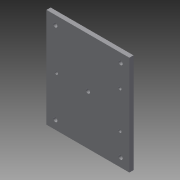
# Autodesk Inventor part: small plate
Saved by Autodesk Inventor 2014 SP1 (Build 180222100, 222)
## iProperties
Created: 2014-02-07
Part Number: small plate
Material: Generic
Document SubType Name: Modeling
Designer: Owner
Density: 1 g/cm^3
Appearance: Default
Author: Owner
Autodesk Inventor part; units mm, degrees
ref_plane "YZ Plane" through (0, 0, 0) normal (1, 0, 0) x (0, 1, 0)
ref_plane "XZ Plane" through (0, 0, 0) normal (0, 1, 0) x (-1, 0, 0)
ref_plane "XY Plane" through (0, 0, 0) normal (0, 0, 1) x (1, 0, 0)
sketch "Sketch1" plane through (0, 0, 0) normal (0, 0, 1) x (1, 0, 0)
  line L0 (-63.5, -76.2) -> (63.5, -76.2)
  line L1 (63.5, -76.2) -> (63.5, 76.2)
  line L2 (63.5, 76.2) -> (-63.5, 76.2)
  line L3 (-63.5, 76.2) -> (-63.5, -76.2)
  line L4 (-63.5, -76.2) -> (63.5, 76.2) construction
  line L5 (63.5, -76.2) -> (-63.5, 76.2) construction
  line L6 (-63.5, 76.2) -> (-50.0296, 62.7296)
  line L7 (-63.5, 76.2) -> (-44.45, 76.2) construction
  line L8 (63.5, 76.2) -> (69.85, 76.2) construction
  line L9 (63.5, 76.2) -> (50.0296, 62.7296)
  line L10 (63.5, -76.2) -> (50.0296, -62.7296)
  line L11 (-63.5, -76.2) -> (-50.0296, -62.7296)
  circle A0 centre (-50.0296, 62.7296) radius 3.175
  circle A1 centre (50.0296, 62.7296) radius 3.175
  circle A2 centre (50.0296, -62.7296) radius 3.175
  circle A3 centre (-50.0296, -62.7296) radius 3.175
  circle A4 centre (0, 0) radius 3.175
  line L12 (0, 0) -> (-48.4, 0) construction
  line L13 (0, 0) -> (3.175, 0)
  line L14 (0, 0) -> (49, 0) construction
  line L15 (49, 0) -> (49, 28.29) construction
  line L16 (49, 0) -> (49, -28.29) construction
  circle A5 centre (49, -28.29) radius 2.4
  circle A6 centre (49, 28.29) radius 2.4
  circle A7 centre (-48.4, 0) radius 2.4
  dimension "d10" = 6.35
  dimension "d0" = 127
  dimension "d1" = 152.4
  dimension "d2" = 19.05
  dimension "d3" = 45
  dimension "d6" = 6.35
  dimension "d7" = 6.35
  dimension "d8" = 6.35
  dimension "d9" = 6.35
  dimension "d11" = 48.4
  dimension "d12" = 49
  dimension "d13" = 28.29
  dimension "d14" = 28.29
  dimension "d15" = 4.8
  dimension "d16" = 4.8
  dimension "d17" = 4.8
  constraints: 34 end point, 8 coincident, 7 centre point, 5 perpendicular, 3 horizontal, 3 parallel, 2 collinear, 2 midpoint, 1 equal length, 1 horizontal alignment, 2 other
  measures "d0" distance of L2.end L1.end
  measures "d1" distance of L1.end L0.end
  measures "d2" distance of L2.end L6.end
  measures "d3" angle of L6 L7
  measures "d6" diameter of A0
  measures "d7" diameter of A1
  measures "d8" diameter of A2
  measures "d9" diameter of A3
  measures "d11" distance of L12.start L12.end
  measures "d12" distance of L12.start L14.end
  measures "d13" distance of L14.end L15.end
  measures "d14" distance of L14.end L16.end
  measures "d15" diameter of A5
  measures "d16" diameter of A6
  measures "d17" diameter of A7
extrude "Extrusion1" add sketch "Sketch1" along normal blind 6.35
body "Solid1"
